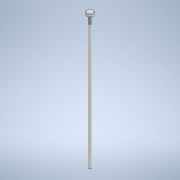
# Autodesk Inventor part: Шуп масло
Saved by Autodesk Inventor 2021 (Build 250183000, 183)
## iProperties
Created: 2023-04-03
Part Number: Шуп масло
Material: Типовые
Document SubType Name: Modeling
Designer: gdevc
Density: 1 g/cm^3
Appearance: По умолчанию
Author: gdevc
Autodesk Inventor part; units mm, degrees
ref_plane "YZ Plane" through (0, 0, 0) normal (1, 0, 0) x (0, 1, 0)
ref_plane "XZ Plane" through (0, 0, 0) normal (0, 1, 0) x (-1, 0, 0)
ref_plane "XY Plane" through (0, 0, 0) normal (0, 0, 1) x (1, 0, 0)
sketch "Эскиз1" plane through (0, 0, 0) normal (0, 0, 1) x (1, 0, 0)
  line L0 (-3, 300) -> (-3, 0)
  line L1 (-3, 0) -> (3, 0)
  line L2 (-3, 306) -> (-7.5, 306)
  line L3 (-7.5, 300) -> (-7.5, 306)
  line L4 (-7.5, 300) -> (-3, 300)
  line L5 (0, 0) -> (0, 306)
  line L6 (0, 306) -> (-3, 306)
  point P0 (0, 300)
  dimension "d1" = 3
  dimension "d4" = 7.5
  dimension "d6" = 6
  dimension "d8" = 300
  constraints: 14 end point, 2 horizontal, 1 collinear, 1 midpoint, 1 parallel, 1 perpendicular, 1 point on line, 1 vertical
  measures "d1" distance from line of L5.start L0
  measures "d4" distance from line of L5.start L3
  measures "d6" distance between parallel lines of L4 L2
  measures "d8" vertical distance of L5.start L0.start
revolve "Вращение1" add sketch "Эскиз1" angle 360 about axis through (0, 0, 0) along (0, 1, 0)
chamfer "Фаска1" distance 1 angle 45 1 edges at (3, 0, 0)
chamfer "Фаска2" distance 1 angle 45 2 edges at (7.5, 306, 0) (7.5, 300, 0)
thread "Резьба1" size "M6x1" class "6g" standard "ISO Metric profile" length 18
equation "\"d1\" = 0.5 * d0"
equation "\"d4\" = 0.5 * d3"
equation "\"d0\" = 6"
equation "\"d3\" = 15"
